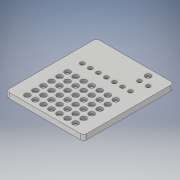
# Autodesk Inventor part: Top Part
Saved by Autodesk Inventor 2018.3 (Build 223284000, 284)
## iProperties
Created: 2019-10-06
Part Number: Top Part
Material: Generic
Document SubType Name: Modeling
Designer: Jamal Bouajjaj
Density: 1 g/cm^3
Appearance: Default
Author: Jamal Bouajjaj
Autodesk Inventor part; units mm, degrees
ref_plane "YZ Plane" through (0, 0, 0) normal (1, 0, 0) x (0, 1, 0)
ref_plane "XZ Plane" through (0, 0, 0) normal (0, 1, 0) x (-1, 0, 0)
ref_plane "XY Plane" through (0, 0, 0) normal (0, 0, 1) x (1, 0, 0)
sketch "Sketch1" plane through (0, 0, 0) normal (0, 1, 0) x (-1, 0, 0)
  line L0 (-2.54, -83.185) -> (-71.12, -83.185) construction
  line L1 (-71.12, -83.185) -> (-71.12, -2.54) construction
  line L2 (-71.12, -2.54) -> (-2.54, -2.54) construction
  line L3 (-2.54, -2.54) -> (-2.54, -83.185) construction
  line L4 (0, -85.725) -> (-73.66, -85.725)
  line L5 (-73.66, -85.725) -> (-73.66, 0)
  line L6 (-73.66, 0) -> (0, 0)
  line L7 (0, 0) -> (0, -85.725)
  line L8 (-2.54, -83.185) -> (0, -85.725) construction
  line L9 (-71.12, -83.185) -> (-73.66, -85.725) construction
  line L10 (-73.66, 0) -> (-71.12, -2.54) construction
  line L11 (-2.54, -2.54) -> (0, 0) construction
  line L12 (-1.5, -84.225) -> (-72.16, -84.225)
  line L13 (-72.16, -84.225) -> (-72.16, -1.5)
  line L14 (-72.16, -1.5) -> (-1.5, -1.5)
  line L15 (-1.5, -1.5) -> (-1.5, -84.225)
  circle A0 centre (-8.255, -79.375) radius 1.6
  circle A1 centre (-65.405, -79.375) radius 1.6
  circle A2 centre (-6.35, -6.35) radius 1.6
  circle A3 centre (-67.31, -6.35) radius 1.6
  line L16 (-8.255, -79.375) -> (-65.405, -79.375) construction
  line L17 (-67.31, -6.35) -> (-6.35, -6.35) construction
  line L18 (-6.35, -6.35) -> (-8.255, -79.375) construction
  line L19 (-65.405, -79.375) -> (-67.31, -6.35) construction
  circle A4 centre (-8.255, -79.375) radius 2.5
  circle A5 centre (-65.405, -79.375) radius 2.5
  circle A6 centre (-67.31, -6.35) radius 2.5
  circle A7 centre (-6.35, -6.35) radius 2.5
  point P0 (0, 0)
  dimension "d0" = 68.58
  dimension "d1" = 80.645
  dimension "d2" = 2.54
  dimension "d3" = 2.54
  dimension "d4" = 1.5
  dimension "d5" = 57.15
  dimension "d6" = 60.96
  dimension "d7" = 73.025
  dimension "d9" = 3.81
  dimension "d10" = 3.81
  dimension "d11" = 3.81
  dimension "d12" = 3.2
  dimension "d13" = 5
  constraints: 40 end point, 8 centre point, 6 equal radius, 6 parallel, 5 coincident, 5 horizontal, 4 equal length, 3 perpendicular, 3 point on line
  measures "d0" distance of L0.start L0.end
  measures "d1" distance of L2.end L0.start
  measures "d2" horizontal distance of L0.start L4.start
  measures "d3" horizontal distance of L0.start L4.start
  measures "d4" distance between parallel lines of L6 L14
  measures "d5" distance of L16.start L16.end
  measures "d6" distance of L17.start L17.end
  measures "d7" vertical distance of L17.end L16.start
  measures "d9" distance from line of L2 L17.end
  measures "d10" vertical distance of L16.start L0.start
  measures "d11" horizontal distance of L2.end L17.end
  measures "d12" diameter of A0
  measures "d13" diameter of A4
extrude "Extrusion1" add sketch "Sketch1" along normal blind 2.54 contours L4 L5 L6 L7 | L12 L13 L14 L15 | A0 | A1 | A2 | A3 | A4 | A5 | A6 | A7
extrude "Extrusion2" add sketch "Sketch1" against normal blind 2.54
sketch "Sketch2" plane through (0, 0, 0) normal (0, -1, 0) x (1, 0, 0)
  circle A0 centre (67.31, -6.35) radius 2.5 projected
  circle A1 centre (8.255, -79.375) radius 2.5 projected
  line L0 (1.5, -1.5) -> (1.5, -84.225) projected
  line L1 (1.5, -84.225) -> (72.16, -84.225) projected
  line L2 (72.16, -84.225) -> (72.16, -1.5) projected
  line L3 (72.16, -1.5) -> (1.5, -1.5) projected
  circle A2 centre (65.405, -79.375) radius 2.5 projected
  circle A3 centre (6.35, -6.35) radius 2.5 projected
  circle A4 centre (59.69, -6.35) radius 2.65
  circle A5 centre (59.69, -13.97) radius 2.65
  circle A6 centre (59.69, -21.59) radius 2.65
  circle A7 centre (59.69, -29.21) radius 2.65
  circle A8 centre (59.69, -36.83) radius 2.65
  circle A9 centre (59.69, -44.45) radius 2.65
  circle A10 centre (52.07, -6.35) radius 2.65
  circle A11 centre (52.07, -13.97) radius 2.65
  circle A12 centre (52.07, -21.59) radius 2.65
  circle A13 centre (52.07, -29.21) radius 2.65
  circle A14 centre (52.07, -36.83) radius 2.65
  circle A15 centre (52.07, -44.45) radius 2.65
  circle A16 centre (44.45, -6.35) radius 2.65
  circle A17 centre (44.45, -13.97) radius 2.65
  circle A18 centre (44.45, -21.59) radius 2.65
  circle A19 centre (44.45, -29.21) radius 2.65
  circle A20 centre (44.45, -36.83) radius 2.65
  circle A21 centre (44.45, -44.45) radius 2.65
  circle A22 centre (36.83, -6.35) radius 2.65
  circle A23 centre (36.83, -13.97) radius 2.65
  circle A24 centre (36.83, -21.59) radius 2.65
  circle A25 centre (36.83, -29.21) radius 2.65
  circle A26 centre (36.83, -36.83) radius 2.65
  circle A27 centre (36.83, -44.45) radius 2.65
  circle A28 centre (29.21, -6.35) radius 2.65
  circle A29 centre (29.21, -13.97) radius 2.65
  circle A30 centre (29.21, -21.59) radius 2.65
  circle A31 centre (29.21, -29.21) radius 2.65
  circle A32 centre (29.21, -36.83) radius 2.65
  circle A33 centre (29.21, -44.45) radius 2.65
  circle A34 centre (21.59, -6.35) radius 2.65
  circle A35 centre (21.59, -13.97) radius 2.65
  circle A36 centre (21.59, -21.59) radius 2.65
  circle A37 centre (21.59, -29.21) radius 2.65
  circle A38 centre (21.59, -36.83) radius 2.65
  circle A39 centre (21.59, -44.45) radius 2.65
  circle A40 centre (13.97, -6.35) radius 2.65
  circle A41 centre (13.97, -13.97) radius 2.65
  circle A42 centre (13.97, -21.59) radius 2.65
  circle A43 centre (13.97, -29.21) radius 2.65
  circle A44 centre (13.97, -36.83) radius 2.65
  circle A45 centre (13.97, -44.45) radius 2.65
  circle A46 centre (59.69, -58.3946) radius 2
  circle A47 centre (52.07, -58.3946) radius 2
  circle A48 centre (44.45, -58.3946) radius 2
  circle A49 centre (36.83, -58.3946) radius 2
  circle A50 centre (29.21, -58.3946) radius 2
  circle A51 centre (21.59, -58.3946) radius 2
  circle A52 centre (13.97, -58.3946) radius 2
  line L4 (67.31, -6.35) -> (59.69, -6.35) construction
  line L5 (65.405, -79.375) -> (59.69, -58.3946) construction
  line L6 (13.97, -58.3946) -> (8.255, -79.375) construction
  circle A53 centre (55.499, -79.375) radius 2.65
  line L7 (55.499, -79.375) -> (65.405, -79.375) construction
  circle A54 centre (55.499, -71.1454) radius 2
  circle A55 centre (63.754, -71.1454) radius 2
  line L8 (55.499, -71.1454) -> (63.754, -71.1454) construction
  line L9 (55.499, -71.1454) -> (55.499, -79.375) construction
  point P0 (0, 0)
  dimension "d20" = 7.62
  dimension "d23" = 7.62
  dimension "d26" = 5.3
  dimension "d29" = 7.62
  dimension "d34" = 7.62
  dimension "d35" = 7.62
  dimension "d36" = 60.96
  dimension "d37" = 20.9804
  dimension "d38" = 4
  dimension "d40" = 9.906
  dimension "d41" = 8.255
  dimension "d42" = 8.2296
  constraints: 52 centre point, 12 end point, 5 horizontal, 3 equal radius, 2 vertical, 1 equal length, 94 other
  measures "d20" distance of L4.end A5.centre
  measures "d23" distance of L4.end A10.centre
  measures "d26" diameter of A4
  measures "d29" distance of L5.end A47.centre
  measures "d34" distance of L4.start L4.end
  measures "d35" distance of A3.centre A40.centre
  measures "d36" distance of A3.centre L4.start
  measures "d37" vertical distance of L5.start L5.end
  measures "d38" diameter of A46
  measures "d40" distance of L7.start L5.start
  measures "d41" distance of L8.start L8.end
  measures "d42" distance of L8.start L7.start
extrude "Extrusion3" cut sketch "Sketch2" against normal through all contours A4 | A5 | A6 | A7 | A8 | A9 | A10 | A11 | A12 | A13 | A14 | A15 | A16 | A17 | A18 | A19 | A20 | A21 | A22 | A23 | A24 | A25 | A26 | A27 | A28 | A29 | A30 | A31 | A32 | A33 | A34 | A35 | A36 | A37 | A38 | A39 | A40 | A41 | A42 | A43 | A44 | A45 | A46 | A47 | A48 | A49 | A50 | A51 | A52 | A53 | A54 | A55
sketch "Sketch3" plane through (0, 0, 0) normal (0, -1, 0) x (1, 0, 0)
  line L0 (1.5, -1.5) -> (1.5, -84.225) projected
  line L1 (1.5, -75.4634) -> (0, -75.4634)
  line L2 (0, -75.4634) -> (0, -66.7512)
  line L3 (0, -66.7512) -> (1.5, -66.7512)
  line L4 (1.5, -66.7512) -> (1.5, -75.4634)
  line L5 (0, -85.725) -> (73.66, -85.725) projected
  line L6 (2.54, -83.185) -> (71.12, -83.185) construction
  line L7 (2.54, -2.54) -> (2.54, -83.185) construction
  line L8 (1.5, -75.4634) -> (4.04, -75.4634)
  line L9 (4.04, -75.4634) -> (4.04, -76.9874)
  line L10 (4.04, -76.9874) -> (1.5, -76.9874)
  line L11 (1.5, -76.9874) -> (1.5, -75.4634)
  line L12 (1.5, -66.7512) -> (4.04, -66.7512)
  line L13 (4.04, -66.7512) -> (4.04, -65.2272)
  line L14 (4.04, -65.2272) -> (1.5, -65.2272)
  line L15 (1.5, -65.2272) -> (1.5, -66.7512)
  line L16 (4.04, -66.7512) -> (4.04, -75.4634) construction
  point P0 (0, 0)
  dimension "d46" = 8.7122
  dimension "d49" = 7.7216
  dimension "d50" = 1.524
  dimension "d53" = 2.54
  constraints: 26 end point, 6 parallel, 3 horizontal, 3 perpendicular, 1 collinear, 1 point on line, 1 vertical
  measures "d46" distance of L1.end L2.end
  measures "d49" distance between parallel lines of L1 L6
  measures "d50" distance of L8.end L9.end
  measures "d53" distance of L1.start L8.end
extrude "Extrusion4" cut sketch "Sketch3" along normal through all contours L0 L1 L2 L3
extrude "Extrusion5" add sketch "Sketch3" along normal up to surface (2.54 mm away) contours L14 L13 L12 L0 | L8 L9 L10 L0
fillet "Fillet1" radius 3.175 8 edges at (1.5, -1.27, -84.225) (0, 0, -85.725) (73.66, 0, -85.725) (72.16, -1.27, -84.225) (72.16, -1.27, -1.5) (73.66, 0, 0) (1.5, -1.27, -1.5) (0, 0, 0)
body "Solid1"
